Autodesk Inventor part; units mm, degrees
(part 2 of 2)
sketch "Sketch28" plane through (0, 126.5801, 132.4443) normal (0, 0.7071068, 0.7071068) x (1, 0, 0)
  line L0 (330, 0) -> (330, -85.314) construction
  line L1 (330, -42.657) -> (0, -42.657) construction
  line L2 (10, 4.1466) -> (10, -123.8398) construction
  circle A0 centre (30, -42.657) radius 11.1
  circle A1 centre (73.2, -42.657) radius 3.2
  circle A2 centre (94.6, -42.657) radius 3.2
  circle A3 centre (116, -42.657) radius 3.2
  circle A4 centre (137.4, -42.657) radius 3.2
  circle A5 centre (158.8, -42.657) radius 3.2
  line L3 (0, -85.314) -> (0, 0)
  circle A6 centre (30, -42.657) radius 20 construction
  line L4 (172, 0) -> (325, 0) construction
  line L5 (325, 0) -> (325, -85.314) construction
  line L6 (325, -85.314) -> (172, -85.314) construction
  line L7 (172, -85.314) -> (172, 0) construction
  line L8 (30, -22.657) -> (158.8, -22.657) construction
  line L9 (73.2, -42.657) -> (73.2, -22.657) construction
  line L10 (94.6, -42.657) -> (94.4, -22.657) construction
  line L11 (116, -42.657) -> (116, -22.657) construction
  line L12 (137.4, -42.657) -> (137.4, -22.657) construction
  line L13 (158.8, -42.657) -> (158.8, -22.657) construction
  line L14 (30, -62.657) -> (158.8, -62.657) construction
  line L15 (73.2, -42.657) -> (73.2, -62.657) construction
  line L16 (94.6, -42.657) -> (94.4, -62.657) construction
  line L17 (116, -42.657) -> (116, -62.657) construction
  line L18 (137.4, -42.657) -> (137.4, -62.657) construction
  line L19 (158.8, -42.657) -> (158.8, -62.657) construction
  circle A7 centre (73.2, -22.657) radius 2.55
  circle A8 centre (94.4, -22.657) radius 2.55
  circle A9 centre (116, -22.657) radius 2.55
  circle A10 centre (137.4, -22.657) radius 2.55
  circle A11 centre (158.8, -22.657) radius 2.55
  circle A12 centre (73.2, -62.657) radius 2.55
  circle A13 centre (94.4, -62.657) radius 2.55
  circle A14 centre (116, -62.657) radius 2.55
  circle A15 centre (137.4, -62.657) radius 2.55
  circle A16 centre (158.8, -62.657) radius 2.55
  line L20 (203.1647, -22.6721) -> (197.1963, -40.7279)
  line L21 (197.1963, -40.7279) -> (203.7374, -62.6721)
  line L22 (203.7374, -62.6721) -> (193.0064, -62.6721)
  line L23 (193.0064, -62.6721) -> (188.7562, -45.5206)
  line L24 (188.7562, -45.5206) -> (188.7562, -62.6721)
  line L25 (188.7562, -62.6721) -> (178.3568, -62.6721)
  line L26 (178.3568, -62.6721) -> (178.3568, -22.6721)
  line L27 (178.3568, -22.6721) -> (188.7562, -22.6721)
  line L28 (188.7562, -22.6721) -> (188.7562, -38.226)
  line L29 (188.7562, -38.226) -> (193.4284, -22.6721)
  line L30 (193.4284, -22.6721) -> (203.1647, -22.6721)
  line L31 (205.5158, -22.6721) -> (212.8708, -22.6721)
  spline S0 degree 2 poles (212.8708, -22.6721) (220.2257, -22.6721) (225.4405, -23.8175) (228.7261, -28.4897) (228.7261, -33.5839) knots 0 0 0 1 2 3 3 3
  spline S1 degree 2 poles (228.7261, -33.5839) (228.7261, -38.2561) (226.4051, -41.4814) (222.9989, -41.813) knots 0 0 0 1 2 2 2
  spline S2 degree 2 poles (222.9989, -41.813) (226.0735, -42.5666) (228.2136, -45.1288) (228.7261, -47.2689) (228.7261, -52.122) knots 0 0 0 1 2 3 3 3
  line L32 (228.7261, -52.122) -> (228.7261, -62.6721)
  line L33 (228.7261, -62.6721) -> (219.0501, -62.6721)
  line L34 (219.0501, -62.6721) -> (219.0501, -49.3789)
  spline S3 degree 2 poles (219.0501, -49.3789) (219.0501, -46.1838) (218.0554, -44.6465) (215.9152, -44.6465) knots 0 0 0 1 2 2 2
  line L35 (215.9152, -44.6465) -> (215.9152, -62.6721)
  line L36 (215.9152, -62.6721) -> (205.5158, -62.6721)
  line L37 (205.5158, -62.6721) -> (205.5158, -22.6721)
  line L38 (215.9152, -29.5146) -> (215.9152, -38.4068)
  spline S4 degree 2 poles (215.9152, -38.4068) (217.6635, -38.4068) (219.0501, -37.4422) (219.0501, -34.7896) knots 0 0 0 1 2 2 2
  line L39 (219.0501, -34.7896) -> (219.0501, -32.5892)
  spline S5 degree 2 poles (219.0501, -32.5892) (219.0501, -30.6902) (217.6937, -29.5146) (215.9152, -29.5146) knots 0 0 0 1 2 2 2
  spline S6 degree 2 poles (260.1353, -39.9743) (262.396, -40.758) (264.6266, -44.2546) (264.6266, -50.6751) knots 0 0 0 1 2 2 2
  spline S7 degree 2 poles (264.6266, -50.6751) (264.6266, -55.4377) (262.4563, -60.7128) (257.121, -63.4558) (252.931, -63.4558) knots 0 0 0 1 2 3 3 3
  spline S8 degree 2 poles (252.931, -63.4558) (248.1986, -63.4558) (242.8029, -60.2606) (241.0848, -55.6487) (241.0848, -49.9517) knots 0 0 0 1 2 3 3 3
  line L40 (241.0848, -49.9517) -> (241.0848, -46.7866)
  line L41 (241.0848, -46.7866) -> (251.0622, -46.7866)
  line L42 (251.0622, -46.7866) -> (251.0622, -53.2674)
  spline S9 degree 2 poles (251.0622, -53.2674) (251.0622, -55.8597) (251.6952, -57.2765) (252.7502, -57.2765) knots 0 0 0 1 2 2 2
  spline S10 degree 2 poles (252.7502, -57.2765) (253.8956, -57.2765) (254.6492, -55.498) (254.6492, -51.7301) knots 0 0 0 1 2 2 2
  line L43 (254.6492, -51.7301) -> (254.6492, -48.9871)
  spline S11 degree 2 poles (254.6492, -48.9871) (254.6492, -46.6661) (253.6243, -44.556) (251.6047, -43.8929) (248.6809, -43.8326) knots 0 0 0 1 2 3 3 3
  line L44 (248.6809, -43.8326) -> (248.6809, -38.015)
  spline S12 degree 2 poles (248.6809, -38.015) (252.2378, -38.015) (253.8956, -37.4724) (254.6492, -35.6337) (254.6492, -33.7045) knots 0 0 0 1 2 3 3 3
  line L45 (254.6492, -33.7045) -> (254.6492, -31.4739)
  spline S13 degree 2 poles (254.6492, -31.4739) (254.6492, -29.3639) (253.7751, -28.0376) (252.8708, -28.0376) knots 0 0 0 1 2 2 2
  spline S14 degree 2 poles (252.8708, -28.0376) (251.8158, -28.0376) (251.0622, -29.4543) (251.0622, -31.7452) knots 0 0 0 1 2 2 2
  line L46 (251.0622, -31.7452) -> (251.0622, -35.0308)
  line L47 (251.0622, -35.0308) -> (241.0848, -35.0308)
  line L48 (241.0848, -35.0308) -> (241.0848, -31.6246)
  spline S15 degree 2 poles (241.0848, -31.6246) (241.0848, -25.8974) (246.3297, -21.8582) (252.0268, -21.8582) knots 0 0 0 1 2 2 2
  spline S16 degree 2 poles (252.0268, -21.8582) (259.1707, -21.8582) (264.2649, -27.4347) (264.2649, -32.4083) knots 0 0 0 1 2 2 2
  spline S17 degree 2 poles (264.2649, -32.4083) (264.2649, -35.7542) (262.4262, -38.7685) (260.1353, -39.9743) knots 0 0 0 1 2 2 2
  line L49 (290.0072, -22.6721) -> (290.0072, -29.0624)
  line L50 (290.0072, -29.0624) -> (277.6183, -29.0624)
  line L51 (277.6183, -29.0624) -> (277.6183, -35.8748)
  spline S18 degree 2 poles (277.6183, -35.8748) (279.9393, -33.1318) (283.6168, -33.1318) knots 0 0 0 1 1 1
  spline S19 degree 2 poles (283.6168, -33.1318) (287.7464, -33.1318) (291.9665, -37.7437) (291.9665, -44.3149) knots 0 0 0 1 2 2 2
  line L52 (291.9665, -44.3149) -> (291.9665, -50.0119)
  spline S20 degree 2 poles (291.9665, -50.0119) (291.9665, -54.2621) (291.1526, -58.241) (288.4699, -61.6171) (283.7072, -63.4257) (280.2709, -63.4257) knots 0 0 0 1 2 3 4 4 4
  spline S21 degree 2 poles (280.2709, -63.4257) (276.4126, -63.4257) (270.5347, -60.7429) (268.0629, -55.4076) (268.0629, -49.8311) knots 0 0 0 1 2 3 3 3
  line L53 (268.0629, -49.8311) -> (268.0629, -47.6608)
  line L54 (268.0629, -47.6608) -> (278.0403, -47.6608)
  line L55 (278.0403, -47.6608) -> (278.0403, -50.1627)
  spline S22 degree 2 poles (278.0403, -50.1627) (278.0403, -54.021) (278.5829, -57.2765) (280.2106, -57.2765) knots 0 0 0 1 2 2 2
  spline S23 degree 2 poles (280.2106, -57.2765) (280.9341, -57.2765) (281.8685, -56.342) (281.9288, -55.2569) (281.9891, -51.067) knots 0 0 0 1 2 3 3 3
  line L56 (281.9891, -51.067) -> (281.9891, -43.1694)
  spline S24 degree 2 poles (281.9891, -43.1694) (281.9891, -40.9087) (281.0546, -39.281) (279.9393, -39.281) knots 0 0 0 1 2 2 2
  spline S25 degree 2 poles (279.9393, -39.281) (279.246, -39.281) (278.3116, -40.125) (278.0403, -41.0896) (278.0403, -42.8379) knots 0 0 0 1 2 3 3 3
  line L57 (278.0403, -42.8379) -> (268.1534, -42.8379)
  line L58 (268.1534, -42.8379) -> (268.5754, -22.6721)
  line L59 (268.5754, -22.6721) -> (290.0072, -22.6721)
  line L60 (318.9145, -36.2064) -> (318.9145, -49.5297)
  spline S26 degree 2 poles (318.9145, -49.5297) (318.9145, -54.0813) (317.9197, -58.241) (314.815, -61.8582) (310.4141, -63.4257) (307.7012, -63.4257) knots 0 0 0 1 2 3 4 4 4
  spline S27 degree 2 poles (307.7012, -63.4257) (304.1142, -63.4257) (299.3817, -61.7678) (296.5482, -58.2712) (295.3726, -54.3827) (295.3726, -50.1627) knots 0 0 0 1 2 3 4 4 4
  line L61 (295.3726, -50.1627) -> (295.3726, -36.2064)
  spline S28 degree 2 poles (295.3726, -36.2064) (295.3726, -30.6902) (297.2717, -25.2041) (302.9386, -21.8884) (306.9476, -21.8884) knots 0 0 0 1 2 3 3 3
  spline S29 degree 2 poles (306.9476, -21.8884) (310.2332, -21.8884) (315.4179, -24.1792) (318.0102, -27.495) (318.9145, -31.6548) (318.9145, -36.2064) knots 0 0 0 1 2 3 4 4 4
  spline S30 degree 2 poles (308.9371, -32.8303) (308.9371, -29.6352) (308.3041, -28.0376) (307.1888, -28.0376) knots 0 0 0 1 2 2 2
  spline S31 degree 2 poles (307.1888, -28.0376) (306.0735, -28.0376) (305.35, -29.7557) (305.35, -32.8303) knots 0 0 0 1 2 2 2
  line L62 (305.35, -32.8303) -> (305.35, -52.3631)
  spline S32 degree 2 poles (305.35, -52.3631) (305.35, -55.8296) (306.0132, -57.2765) (307.1285, -57.2765) knots 0 0 0 1 2 2 2
  spline S33 degree 2 poles (307.1285, -57.2765) (308.2438, -57.2765) (308.9371, -55.5884) (308.9371, -52.6645) knots 0 0 0 1 2 2 2
  line L63 (308.9371, -52.6645) -> (308.9371, -32.8303)
  point P0 (0, 4.1466)
  point P1 (0, 4.1466)
  dimension "d182" = 40
  dimension "d175" = 22.2
  dimension "d176" = 6.4
  dimension "d177" = 6.4
  dimension "d178" = 6.4
  dimension "d179" = 6.4
  dimension "d180" = 6.4
  dimension "d181" = 30
  dimension "d183" = 43.2
  dimension "d184" = 21.4
  dimension "d185" = 21.4
  dimension "d186" = 21.4
  dimension "d187" = 21.4
  dimension "d188" = 10
  dimension "d189" = 13.2
  dimension "d190" = 0
  dimension "d191" = 0
  dimension "d192" = 5.1
  dimension "d193" = 5.1
  dimension "d194" = 5.1
  dimension "d195" = 5.1
  dimension "d196" = 5.1
  constraints: 32 end point, 16 centre point, 12 point on line, 11 symmetric about line, 6 coincident, 6 perpendicular, 2 midpoint, 1 horizontal, 1 vertical alignment, 9 other
  measures "d175" diameter of A0
  measures "d176" diameter of A1
  measures "d177" diameter of A2
  measures "d178" diameter of A3
  measures "d179" diameter of A4
  measures "d180" diameter of A5
  measures "d181" distance from line of L3 A0.centre
  measures "d183" distance of L9.start point (30, -42.657)
  measures "d184" distance of L9.start L10.start
  measures "d185" distance of L11.start L10.start
  measures "d186" distance of L11.start L12.start
  measures "d187" distance of L12.start L13.start
  measures "d188" diameter of L5 L0
  measures "d189" distance from line of L13.start L7
  measures "d190" distance from line of L0.start L4
  measures "d191" distance from line of L0.end L6
  measures "d192" diameter of A7
  measures "d193" diameter of A8
  measures "d194" diameter of A9
  measures "d195" diameter of A10
  measures "d196" diameter of A11
emboss "Emboss1" sketch "Sketch28" operation cut depth 1 direction (0, -0.7071068, -0.7071068) contours L20 L21 L22 L23 L24 L25 L26 L27 L28 L29 L30 | L31 S0 S1 S2 L32 L33 L34 S3 L35 L36 L37 | S6 S7 S8 L40 L41 L42 S9 S10 L43 S11 L44 S12 L45 S13 S14 L46 L47 L48 S15 S16 S17 | L49 L50 L51 S18 S19 L52 S20 S21 L53 L54 L55 S22 S23 L56 S24 S25 L57 L58 L59 | L60 S26 S27 L61 S28 S29
ref_plane "Work Plane1" through (60, 0, 0) normal (1, 0, 0) x (0, 0, -1)
sketch "Sketch29" plane through (60, 0, 0) normal (1, 0, 0) x (0, 0, -1)
  circle A0 centre (-109.0443, 122.0272) radius 2.1 projected
  line L0 (-109.0443, 122.0272) -> (-109.0443, 0.25) construction
  line L1 (-1, 0.25) -> (-178, 0.25) projected
  line L2 (3, 116.0545) -> (-129.0164, 116.0545) projected
  line L3 (-112.0443, 116.0545) -> (-106.0443, 116.0545)
  line L4 (-106.0443, 116.0545) -> (-106.0443, 106.0545)
  line L5 (-106.0443, 106.0545) -> (-112.0443, 106.0545)
  line L6 (-112.0443, 106.0545) -> (-112.0443, 116.0545)
  point P0 (0, 0)
  dimension "d201" = 6
  dimension "d202" = 10
  dimension "d203" = 3
  constraints: 10 end point, 2 parallel, 2 point on line, 1 horizontal, 1 perpendicular, 1 vertical
  measures "d201" distance of L4.end L5.end
  measures "d202" distance of L3.end L4.end
  measures "d203" distance between parallel lines of L0 L4
extrude "Extrusion26" add sketch "Sketch29" along normal blind 10 contours L4 L5 L6 L2
ref_plane "Work Plane2" through (170, 0, 0) normal (1, 0, 0) x (0, 0, -1)
sketch "Sketch30" plane through (170, 0, 0) normal (1, 0, 0) x (0, 0, -1)
  line L0 (-112.0443, 116.0545) -> (-112.0443, 106.0545) projected
  line L1 (-112.0443, 106.0545) -> (-106.0443, 106.0545) projected
  line L2 (-106.0443, 106.0545) -> (-106.0443, 116.0545) projected
  line L3 (-112.0443, 116.0545) -> (-106.0443, 116.0545) projected
  point P0 (0, 0)
extrude "Extrusion27" add sketch "Sketch30" along normal blind 10
ref_plane "Work Plane3" through (276, 0, 0) normal (1, 0, 0) x (0, 0, -1)
sketch "Sketch31" plane through (276, 0, 0) normal (1, 0, 0) x (0, 0, -1)
  line L0 (-112.0443, 116.0545) -> (-112.0443, 106.0545) projected
  line L1 (-112.0443, 106.0545) -> (-106.0443, 106.0545) projected
  line L2 (-106.0443, 106.0545) -> (-106.0443, 116.0545) projected
  line L3 (-112.0443, 116.0545) -> (-106.0443, 116.0545) projected
  point P0 (0, 0)
extrude "Extrusion28" add sketch "Sketch31" along normal blind 10
sketch "Sketch32" plane through (276, 106.0545, 106.0443) normal (0, 0, -1) x (-1, 0, 0)
  line L0 (-10, 10) -> (-10, 0) construction
  line L1 (7.4246, 4.4941) -> (-14.0072, 4.4941) construction
  line L2 (96, 0) -> (96, 10) construction
  line L3 (96, 5) -> (106, 5) construction
  line L4 (106, 0) -> (106, 10) construction
  line L5 (206, 10) -> (206, 0) construction
  line L6 (206, 5) -> (216, 5) construction
  line L7 (216, 0) -> (216, 10) construction
  line L8 (-10, 5) -> (0, 5) construction
  line L9 (0, 10) -> (0, 0) construction
  circle A0 centre (-5, 5) radius 3
  circle A1 centre (101, 5) radius 3
  circle A2 centre (211, 5) radius 3
  point P0 (276, -106.0545)
  dimension "d212" = 6
  dimension "d213" = 6
  dimension "d214" = 6
  constraints: 9 midpoint, 6 end point, 3 centre point
  measures "d212" diameter of A0
  measures "d213" diameter of A1
  measures "d214" diameter of A2
extrude "Extrusion29" cut sketch "Sketch32" against normal up to next
chamfer "Chamfer3" distance 10 angle 45 3 edges at (276, 116.0545, 109.0443) (170, 116.0545, 109.0443) (60, 116.0545, 109.0443)
sketch "Sketch33" plane through (0, 128, 127.4396) normal (0, 1, 0) x (1, 0, 0)
  line L0 (0, 130.4396) -> (320, 130.4396) construction
  line L1 (320, 130.4396) -> (0, 130.4396) construction
  line L2 (0, 130.4396) -> (0, 0) construction
  line L3 (0, 0) -> (320, 0) construction
  line L4 (320, 0) -> (320, 130.4396) construction
  line L5 (0, 130.4396) -> (0, 0) construction
  line L6 (0, 65.2198) -> (320, 65.2198) construction
  line L7 (320, -1.5768) -> (320, 130.4396) construction
  line L8 (197.9145, 39.2198) -> (197.9145, 91.2198)
  line L9 (197.9145, 39.2198) -> (265.1344, 39.2198)
  line L10 (265.1344, 91.2198) -> (197.9145, 91.2198)
  line L11 (197.9145, 91.2198) -> (197.9145, 39.2198)
  arc A0 (265.1344, 39.2198) -> (265.1344, 91.2198) centre (272.4145, 65.2198) ccw
  arc A1 (265.1344, 39.2198) -> (265.1344, 91.2198) centre (272.4145, 65.2198) ccw
  line L12 (318.9145, -30.6065) -> (318.9145, -40.0275) construction
  line L13 (198.0843, 38.9698) -> (265.1001, 38.9698)
  arc A2 (265.1001, 38.9698) -> (265.1001, 91.4698) centre (272.4145, 65.2198) ccw
  line L14 (265.1001, 91.4698) -> (198.2137, 91.4698)
  line L15 (197.6645, 38.7323) -> (197.6645, 90.7321)
  line L16 (197.6645, 90.7321) -> (197.6645, 91.4698)
  line L17 (197.6645, 91.4698) -> (198.2137, 91.4698)
  line L18 (197.6645, 38.7323) -> (197.6645, 38.9698)
  line L19 (197.6645, 38.9698) -> (198.0843, 38.9698)
  point P0 (0, 127.4396)
  dimension "d299" = 27
  dimension "d300" = 67.2199
  dimension "d301" = 67.2199
  dimension "d302" = 52
  dimension "d303" = 74.5
  dimension "d304" = 26
  dimension "d305" = 26
  dimension "d306" = 121
  dimension "d307" = 0.25
  dimension "d308" = 0.25
  dimension "d309" = 0.25
  dimension "d310" = 0.25
  constraints: 32 end point, 6 parallel, 6 point on circle, 3 centre point, 2 perpendicular, 1 coincident, 1 collinear, 1 horizontal, 1 midpoint, 1 point on line, 1 vertical
  measures "d299" radius of A1
  measures "d300" distance of L8.start L9.end
  measures "d301" distance of L10.start L8.end
  measures "d302" distance of L8.start L8.end
  measures "d303" distance from line of L8 A1.centre
  measures "d304" distance from line of L9 A1.centre
  measures "d305" distance between parallel lines of L6 L10
  measures "d306" distance from line of L8 L12.start
  measures "d307" distance between parallel lines of L9 L13
  measures "d308" radial gap between concentric circles of A0 A2
  measures "d309" distance between parallel lines of L10 L14
  measures "d310" distance between parallel lines of L8 L15
extrude "Extrusion30" cut sketch "Sketch33" against normal blind 3.5 contours L8 L10 A0 L9 | L19 L15 L16 L17 L14 A2 L13
sketch "Sketch34" plane through (0, 124.5, 127.4396) normal (0, 1, 0) x (1, 0, 0)
  line L0 (230.4145, 148.8787) -> (230.4145, -93.6412)
  line L1 (197.6645, 38.9698) -> (197.6645, 91.4698) projected
  line L2 (197.6645, 91.4698) -> (265.1001, 91.4698) projected
  line L3 (197.6645, 38.9698) -> (197.6645, 91.4698) projected
  line L4 (265.1001, 38.9698) -> (197.6645, 38.9698) projected
  arc A0 (265.1001, 38.9698) -> (265.1001, 91.4698) centre (272.4145, 65.2198) ccw projected
  line L5 (0, 92) -> (7, 92)
  line L6 (0, 92) -> (0, 0)
  line L7 (0, 0) -> (7, 0)
  arc A1 (7, 0) -> (42, 14) centre (7, 50.75) ccw
  arc A2 (42, 14) -> (42, 78) centre (-127.1667, 46) ccw
  arc A3 (42, 78) -> (7, 92) centre (7, 41.25) ccw
  arc A4 (37.385, 75.4526) -> (7, 87) centre (7, 41.25) ccw
  arc A5 (37.385, 16.5474) -> (37.385, 75.4526) centre (-127.1667, 46) ccw
  arc A6 (7, 5) -> (37.385, 16.5474) centre (7, 50.75) ccw
  line L8 (5, 5) -> (7, 5)
  line L9 (5, 87) -> (5, 5)
  line L10 (5, 87) -> (7, 87)
  point P0 (0, 127.4396)
  point P1 (230.4145, 91.4698)
  point P2 (230.4145, 38.9698)
  point P3 (0, -26.3)
  dimension "d313" = 32.75
  constraints: 14 end point, 12 point on circle, 6 centre point, 1 vertical
  measures "d313" distance between parallel lines of L1 L0
extrude "Extrusion31" add sketch "Sketch34" along normal blind 2.5 contours L2 A0 L4 L0
sketch "Sketch35" plane through (0, 128, 127.4396) normal (0, 1, 0) x (1, 0, 0)
  line L0 (114, 58.4396) -> (114, 51.4396)
  line L1 (114, 58.4396) -> (22, 58.4396)
  line L2 (22, 58.4396) -> (22, 51.4396)
  arc A0 (22, 51.4396) -> (36, 16.4396) centre (72.75, 51.4396) ccw
  arc A1 (36, 16.4396) -> (100, 16.4396) centre (68, 185.6062) ccw
  arc A2 (100, 16.4396) -> (114, 51.4396) centre (63.25, 51.4396) ccw
  arc A3 (97.4526, 21.0546) -> (109, 51.4396) centre (63.25, 51.4396) ccw
  arc A4 (38.5474, 21.0546) -> (97.4526, 21.0546) centre (68, 185.6062) ccw
  arc A5 (27, 51.4396) -> (38.5474, 21.0546) centre (72.75, 51.4396) ccw
  line L3 (27, 53.4396) -> (27, 51.4396)
  line L4 (109, 53.4396) -> (27, 53.4396)
  line L5 (109, 53.4396) -> (109, 51.4396)
  line L6 (0, 130.4396) -> (320, 130.4396) projected
  line L7 (0, 130.4396) -> (0, 0) projected
  arc A6 (21.85, 51.4396) -> (35.9247, 16.3011) centre (72.75, 51.4396) ccw
  line L8 (21.85, 51.4396) -> (21.85, 58.5896)
  line L9 (21.85, 58.5896) -> (114.15, 58.5896)
  line L10 (114.15, 58.5896) -> (114.15, 51.4396)
  arc A7 (100.0753, 16.3011) -> (114.15, 51.4396) centre (63.25, 51.4396) ccw
  arc A8 (35.9247, 16.3011) -> (100.0753, 16.3011) centre (68, 185.6062) ccw
  point P0 (0, 127.4396)
  dimension "d316" = 72
  dimension "d317" = 92
  dimension "d318" = 82
  dimension "d319" = 167.1667
  dimension "d320" = 45.75
  dimension "d321" = 45.75
  dimension "d322" = 50.75
  dimension "d323" = 172.1667
  dimension "d324" = 50.75
  dimension "d325" = 7
  dimension "d326" = 7
  dimension "d327" = 2
  dimension "d328" = 2
  dimension "d329" = 5
  dimension "d330" = 32.385
  dimension "d331" = 32.385
  dimension "d332" = 22
  dimension "d333" = 0.15
  constraints: 18 end point, 18 point on circle, 9 centre point, 6 perpendicular, 3 concentric, 5 other
  measures "d316" distance between parallel lines of L6 L1
  measures "d317" distance of L0.start L1.end
  measures "d318" distance of L4.start L3.start
  measures "d319" radius of A4
  measures "d320" radius of A3
  measures "d321" radius of A5
  measures "d322" radius of A0
  measures "d323" radius of A1
  measures "d324" radius of A2
  measures "d325" distance of L0.start L0.end
  measures "d326" distance of L1.end L2.end
  measures "d327" distance of L3.start L3.end
  measures "d328" distance of L4.start L5.end
  measures "d329" distance between parallel lines of L1 L4
  measures "d330" distance from line of L4 A4.start
  measures "d331" distance from line of L4 A3.start
  measures "d332" distance between parallel lines of L7 L2
  measures "d333" radial gap between concentric circles of A0 A6
extrude "Extrusion32" cut sketch "Sketch35" against normal blind 5 contours L0 A2 A1 A0 L2 L1 | A4 A5 L3 L4 L5 A3 | L8 L9 L10 A7 A8 A6
sketch "Sketch36" plane through (0, 123, 127.4396) normal (0, 1, 0) x (1, 0, 0)
  line L0 (114, 58.4396) -> (114, 51.4396)
  line L1 (114, 58.4396) -> (22, 58.4396)
  line L2 (22, 58.4396) -> (22, 51.4396)
  arc A0 (22, 51.4396) -> (36, 16.4396) centre (72.75, 51.4396) ccw
  arc A1 (36, 16.4396) -> (100, 16.4396) centre (68, 185.6062) ccw
  arc A2 (100, 16.4396) -> (114, 51.4396) centre (63.25, 51.4396) ccw
  arc A3 (97.4526, 21.0546) -> (109, 51.4396) centre (63.25, 51.4396) ccw
  arc A4 (38.5474, 21.0546) -> (97.4526, 21.0546) centre (68, 185.6062) ccw
  arc A5 (27, 51.4396) -> (38.5474, 21.0546) centre (72.75, 51.4396) ccw
  line L3 (27, 53.4396) -> (27, 51.4396)
  line L4 (109, 53.4396) -> (27, 53.4396)
  line L5 (109, 53.4396) -> (109, 51.4396)
  line L6 (0, 130.4396) -> (320, 130.4396)
  line L7 (0, 130.4396) -> (0, 0)
  arc A6 (21.85, 51.4396) -> (35.9247, 16.3011) centre (72.75, 51.4396) ccw
  line L8 (21.85, 51.4396) -> (21.85, 58.5896)
  line L9 (21.85, 58.5896) -> (114.15, 58.5896)
  line L10 (114.15, 58.5896) -> (114.15, 51.4396)
  arc A7 (100.0753, 16.3011) -> (114.15, 51.4396) centre (63.25, 51.4396) ccw
  arc A8 (35.9247, 16.3011) -> (100.0753, 16.3011) centre (68, 185.6062) ccw
  point P0 (0, 127.4396)
  point P1 (0, 127.4396)
  dimension "d336" = 72
  dimension "d337" = 92
  dimension "d338" = 82
  dimension "d339" = 167.1667
  dimension "d340" = 45.75
  dimension "d341" = 45.75
  dimension "d342" = 50.75
  dimension "d343" = 172.1667
  dimension "d344" = 50.75
  dimension "d345" = 7
  dimension "d346" = 7
  dimension "d347" = 2
  dimension "d348" = 2
  dimension "d349" = 5
  dimension "d350" = 32.385
  dimension "d351" = 32.385
  dimension "d352" = 22
  dimension "d353" = 0.15
  constraints: 22 end point, 18 point on circle, 9 centre point, 6 perpendicular, 3 concentric, 5 other
  measures "d336" distance between parallel lines of L6 L1
  measures "d337" distance of L0.start L1.end
  measures "d338" distance of L4.start L3.start
  measures "d339" radius of A4
  measures "d340" radius of A3
  measures "d341" radius of A5
  measures "d342" radius of A0
  measures "d343" radius of A1
  measures "d344" radius of A2
  measures "d345" distance of L0.start L0.end
  measures "d346" distance of L1.end L2.end
  measures "d347" distance of L3.start L3.end
  measures "d348" distance of L4.start L5.end
  measures "d349" distance between parallel lines of L1 L4
  measures "d350" distance from line of L4 A4.start
  measures "d351" distance from line of L4 A3.start
  measures "d352" distance between parallel lines of L7 L2
  measures "d353" radial gap between concentric circles of A0 A6
extrude "Extrusion33" cut sketch "Sketch36" against normal up to next contours A4 A5 L3 L4 L5 A3
sketch "Sketch37" plane through (0, 128, 127.4396) normal (0, 1, 0) x (1, 0, 0)
  line L0 (21.85, 58.5896) -> (114.15, 58.5896) projected
  line L1 (43, 58.5896) -> (93, 58.5896)
  line L2 (93, 58.5896) -> (93, 71.069)
  line L3 (93, 71.069) -> (43, 71.069)
  line L4 (43, 71.069) -> (43, 58.5896)
  point P0 (0, 127.4396)
  dimension "d356" = 50
  dimension "d357" = 21.15
  constraints: 8 end point, 2 parallel, 1 horizontal, 1 perpendicular, 1 point on line
  measures "d356" distance of L3.end L2.end
  measures "d357" distance from line of L0.end L2
extrude "Extrusion34" add sketch "Sketch37" along normal blind 50
chamfer "Chamfer4" distance 10 distance2 25 1 edges at (68, 128, 56.3706) measured on face at (68, 128, 55.8706)
chamfer "Chamfer5" distance 10 angle 45 2 edges at (93, 178, 62.6103) (43, 178, 62.6103)
sketch "Sketch38" plane through (93, 153, 56.3706) normal (0, 0, -1) x (-1, 0, 0)
  line L0 (50, 0) -> (0, 0) construction
  line L1 (50, 0) -> (0, 0) construction
  line L2 (0, 0) -> (0, 25) construction
  line L3 (0, 25) -> (50, 25) construction
  line L4 (50, 25) -> (50, 0) construction
  line L5 (0, 0) -> (0, 15) construction
  line L6 (0, 12.5) -> (50, 12.5) construction
  line L7 (50, 0) -> (50, 15) construction
  circle A0 centre (10, 12.5) radius 2.75
  circle A1 centre (40, 12.5) radius 2.75
  line L8 (10, 25) -> (40, 25) projected
  line L9 (25, 25) -> (25, 0) construction
  point P0 (93, -153)
  dimension "d366" = 50
  dimension "d367" = 12.5
  dimension "d368" = 5.5
  dimension "d369" = 5.5
  dimension "d370" = 15
  dimension "d371" = 15
  constraints: 12 end point, 4 point on line, 2 centre point, 2 midpoint, 2 parallel, 2 perpendicular, 1 horizontal
  measures "d366" distance of L2.end L3.end
  measures "d367" distance between parallel lines of L0 L6
  measures "d368" diameter of A0
  measures "d369" diameter of A1
  measures "d370" distance from line of L9 A0.centre
  measures "d371" distance from line of L9 A1.centre
extrude "Extrusion35" cut sketch "Sketch38" against normal through all
body "Solid1"
